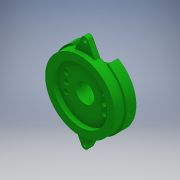
# Autodesk Inventor part: pin_r1
Saved by Autodesk Inventor 2018 (Build 220112000, 112)
## iProperties
Created: 2019-05-28
Part Number: pin_r1
Material: Generic
Document SubType Name: Modeling
Designer: Koki
Density: 1 g/cm^3
Appearance: Dark Green
Author: Koki
Autodesk Inventor part; units mm, degrees
ref_plane "YZ Plane" through (0, 0, 0) normal (1, 0, 0) x (0, 1, 0)
ref_plane "XZ Plane" through (0, 0, 0) normal (0, 1, 0) x (-1, 0, 0)
ref_plane "XY Plane" through (0, 0, 0) normal (0, 0, 1) x (1, 0, 0)
sketch "Sketch1" plane through (0, 0, 0) normal (0, 1, 0) x (-1, 0, 0)
  circle A0 centre (0, 0) radius 10.75
  circle A1 centre (0, 0) radius 13.75
  dimension "d0" = 21.5
  dimension "d1" = 3
  constraints: 2 centre point, 2 coincident
  measures "d0" diameter of A0
  measures "d1" radial gap between concentric circles of A1 A0
extrude "Extrusion1" add sketch "Sketch1" along normal blind 1.9
sketch "Sketch2" plane through (0, 1.9, 0) normal (0, 1, 0) x (1, 0, 0)
  circle A0 centre (0, 0) radius 13.75 projected
extrude "Extrusion2" add sketch "Sketch2" along normal blind 2
sketch "Sketch3" plane through (0, 3.9, 0) normal (0, 1, 0) x (1, 0, 0)
  circle A0 centre (0, 0) radius 1.75
  dimension "d6" = 3.5
  constraints: 1 centre point, 1 coincident
  measures "d6" diameter of A0
extrude "Extrusion3" cut sketch "Sketch3" along normal through all both and the other way through all
sketch "Sketch4" plane through (0, 1.9, 0) normal (0, -1, 0) x (1, 0, 0)
  circle A0 centre (7.5, 0.0066) radius 0.95
  circle A1 centre (7.5, -3.3934) radius 0.95
  circle A2 centre (7.5, 3.4066) radius 0.95
  point P0 (0, 0)
  dimension "d9" = 1.9
  dimension "d10" = 1.9
  dimension "d11" = 1.9
  dimension "d12" = 7.5
  dimension "d13" = 7.5
  dimension "d14" = 7.5
  dimension "d15" = 3.4
  dimension "d16" = 3.4
  constraints: 3 centre point
  measures "d9" diameter of A0
  measures "d10" diameter of A1
  measures "d11" diameter of A2
  measures "d12" distance of point (0, 0) A0.centre
  measures "d13" horizontal distance of point (0, 0) A1.centre
  measures "d14" horizontal distance of point (0, 0) A2.centre
  measures "d15" distance of A0.centre A2.centre
  measures "d16" distance of A1.centre A0.centre
extrude "Extrusion4" [suppressed]
pattern_circular "Circular Pattern1" [suppressed]
sketch "Sketch5" plane through (0, 3.9, 0) normal (0, 1, 0) x (1, 0, 0)
  circle A0 centre (0, -17.85) radius 0.8
  circle A1 centre (0, -17.85) radius 1.45
  circle A2 centre (0, 0) radius 13.75 projected
  line L0 (-1.2939, -18.5046) -> (-4, -13.1553)
  line L1 (1.2939, -18.5046) -> (4, -13.1553)
  dimension "d22" = 1.6
  dimension "d23" = 17.85
  dimension "d24" = 2.9
  dimension "d25" = 0
  dimension "d26" = 4
  dimension "d27" = 4
  constraints: 4 end point, 4 point on circle, 2 centre point, 2 tangent, 1 coincident
  measures "d22" diameter of A0
  measures "d23" distance of point (0, 0) A0.centre
  measures "d24" diameter of A1
  measures "d25" horizontal distance of point (0, 0) A0.centre
  measures "d26" horizontal distance of point (0, 0) L0.end
  measures "d27" horizontal distance of point (0, 0) L1.end
extrude "Extrusion5" add sketch "Sketch5" against normal blind 2 contours A1 | A1 L0 A2 L1
sketch "Sketch6" plane through (0, 3.9, 0) normal (0, 1, 0) x (1, 0, 0)
  circle A0 centre (0, 0) radius 14.35
  dimension "d30" = 28.7
  constraints: 1 centre point, 1 coincident
  measures "d30" diameter of A0
extrude "Extrusion6" add sketch "Sketch6" along normal blind 4
sketch "Sketch7" plane through (0, 7.9, 0) normal (0, 1, 0) x (1, 0, 0)
  circle A0 centre (0, 0) radius 1.75 projected
  line L0 (0, 0) -> (0, -16.57)
  line L1 (0, -16.57) -> (7.1751, -12.4274)
  line L2 (7.1751, -12.4274) -> (0, 0)
  circle A1 centre (0, 0) radius 14.35 projected
  arc A2 (7.1751, -12.4274) -> (-7.1751, -12.4274) centre (0, -16.57) ccw
  arc A3 (-7.1751, -12.4274) -> (7.1751, -12.4274) centre (0, 0) ccw
  dimension "d33" = 16.57
  constraints: 6 end point, 4 point on circle, 2 centre point, 2 coincident, 1 perpendicular, 1 vertical, 3 other
  measures "d33" distance of L0.start L0.end
extrude "Extrusion7" cut sketch "Sketch7" against normal blind 4 contours A2 A1 L0 | L0 A1 A2
sketch "Sketch8" plane through (0, 1.9, 0) normal (0, -1, 0) x (1, 0, 0)
  circle A0 centre (-3.4066, 7.5) radius 0.95 projected
  arc A1 (-7.1751, 12.4274) -> (-6.8562, 11.9187) centre (0, 16.57) ccw projected
  circle A2 centre (-0.0066, 7.5) radius 0.95 projected
  circle A3 centre (3.3934, 7.5) radius 0.95 projected
  circle A4 centre (7.5, 3.4066) radius 0.95 projected
  circle A5 centre (7.5, 0.0066) radius 0.95 projected
  circle A6 centre (7.5, -3.3934) radius 0.95 projected
  circle A7 centre (3.4066, -7.5) radius 0.95 projected
  circle A8 centre (0.0066, -7.5) radius 0.95 projected
  circle A9 centre (-3.3934, -7.5) radius 0.95 projected
  circle A10 centre (-7.5, -3.4066) radius 0.95 projected
  circle A11 centre (-7.5, -0.0066) radius 0.95 projected
  circle A12 centre (-7.5, 3.3934) radius 0.95 projected
  circle A13 centre (0, 0) radius 1.75 projected
  arc A14 (-7.1751, 12.4274) -> (7.1751, 12.4274) centre (0, 0) ccw projected
  arc A15 (6.8562, 11.9187) -> (7.1751, 12.4274) centre (0, 16.57) ccw projected
  arc A16 (-6.8562, 11.9187) -> (6.8562, 11.9187) centre (0, 0) ccw projected
  point P0 (0.5052, 8.3003)
  point P1 (-0.5172, 8.3011)
extrude "Extrusion8" [suppressed]
sketch "Sketch9" plane through (0, 1.9, 0) normal (0, -1, 0) x (1, 0, 0)
  circle A0 centre (0, 0) radius 3.75
  dimension "d38" = 7.5
  constraints: 1 centre point, 1 coincident
  measures "d38" diameter of A0
extrude "Extrusion9" cut sketch "Sketch9" against normal through all
sketch "Sketch10" plane through (0, 1.9, 0) normal (0, -1, 0) x (1, 0, 0)
  circle A0 centre (7.5, 3.4) radius 1.05
  circle A1 centre (7.5, 0) radius 1.05
  circle A2 centre (7.5, -3.4) radius 1.05
  point P0 (0, 0)
  dimension "d41" = 2.1
  dimension "d42" = 2.1
  dimension "d43" = 2.1
  dimension "d44" = 0
  dimension "d45" = 7.5
  dimension "d46" = 7.5
  dimension "d47" = 7.5
  dimension "d48" = 3.4
  dimension "d49" = 3.4
  constraints: 3 centre point
  measures "d41" diameter of A0
  measures "d42" diameter of A1
  measures "d43" diameter of A2
  measures "d44" vertical distance of point (0, 0) A1.centre
  measures "d45" distance of A1.centre point (0, 0)
  measures "d46" horizontal distance of point (0, 0) A2.centre
  measures "d47" horizontal distance of point (0, 0) A0.centre
  measures "d48" distance of A1.centre A0.centre
  measures "d49" distance of A2.centre A1.centre
extrude "Extrusion10" cut sketch "Sketch10" against normal through all
pattern_circular "Circular Pattern2" [suppressed]
pattern_circular "Circular Pattern4" count 2 over 360 about axis through (0, -10, 0) along (0, 1, 0) of "Extrusion10"
sketch "Sketch11" plane through (0, 7.9, 0) normal (0, 1, 0) x (1, 0, 0)
  circle A0 centre (7.5, -3.4) radius 1.05 projected
  circle A1 centre (7.5, 0) radius 1.05 projected
  circle A2 centre (7.5, 3.4) radius 1.05 projected
  circle A3 centre (7.5, -3.4) radius 1.65
  circle A4 centre (7.5, 0) radius 1.65
  circle A5 centre (7.5, 3.4) radius 1.65
  point P0 (0, 0)
  dimension "d61" = 3.3
  dimension "d62" = 3.3
  dimension "d63" = 3.3
  constraints: 3 centre point, 3 coincident
  measures "d61" diameter of A3
  measures "d62" diameter of A4
  measures "d63" diameter of A5
extrude "Extrusion11" cut sketch "Sketch11" against normal blind 3 contours A0 | A1 | A2 | A3 | A4 | A5
pattern_circular "Circular Pattern5" count 2 over 360 about axis through (0, -10, 0) along (0, 1, 0) of "Extrusion11"
pattern_circular "Circular Pattern6" [suppressed]
mirror "Mirror1" about plane through (0, 0, 0) normal (0, 0, 1) of "Extrusion5"
mirror "Mirror2" about plane through (0, 0, 0) normal (0, 0, 1) of "Extrusion7"
equation "\"d13\" = d12"
equation "\"d14\" = d12"
equation "\"d16\" = d15"
equation "\"d27\" = d26"
equation "\"d46\" = d45"
equation "\"d47\" = d45"
equation "\"d49\" = d48"
body "Solid1"
